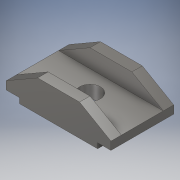
# Autodesk Inventor part: Block2
Saved by Autodesk Inventor 2019 (Build 230136000, 136)
## iProperties
Created: 2018-11-06
Part Number: Block2
Material: Stainless Steel
Document SubType Name: Modeling
Designer: 2003189
Density: 8 g/cm^3
Appearance: Semi-Polished
Mass: 1331.26 g
Surface Area: 349.634 cm^2
Volume: 166.407 cm^3
Author: 2003189
Autodesk Inventor part; units mm, degrees
ref_plane "YZ Plane" through (0, 0, 0) normal (1, 0, 0) x (0, 1, 0)
ref_plane "XZ Plane" through (0, 0, 0) normal (0, 1, 0) x (-1, 0, 0)
ref_plane "XY Plane" through (0, 0, 0) normal (0, 0, 1) x (1, 0, 0)
sketch "Sketch1" plane through (0, 0, 0) normal (0, 0, 1) x (1, 0, 0)
  line L0 (0, 0) -> (127, 0)
  line L1 (127, 0) -> (127, 38.1)
  line L2 (127, 38.1) -> (0, 38.1)
  line L3 (0, 38.1) -> (0, 0)
  line L4 (0, 0) -> (16.129, 0)
  line L5 (127, 0) -> (110.871, 0)
  line L6 (16.129, 0) -> (16.129, 6.35)
  line L7 (16.129, 6.35) -> (0, 6.35)
  line L8 (110.871, 0) -> (110.871, 6.35)
  line L9 (110.871, 6.35) -> (127, 6.35)
  dimension "d0" = 127
  dimension "d1" = 38.1
  dimension "d2" = 16.129
  dimension "d3" = 16.129
  dimension "d4" = 6.35
  dimension "d5" = 6.35
  constraints: 20 end point, 6 point on line, 2 parallel, 2 perpendicular, 1 horizontal, 1 vertical
  measures "d0" distance of L2.end L1.end
  measures "d1" distance of L1.end L0.end
  measures "d2" distance of L0.start L4.end
  measures "d3" distance of L0.end L5.end
  measures "d4" distance of L4.end L6.end
  measures "d5" distance of L5.end L8.end
extrude "Extrusion1" add sketch "Sketch1" along normal blind 76.2 contours L6 L7 L3 L2 L1 L9 L8 L0
chamfer "Chamfer5" distance 38.1 angle 30 2 edges at (127, 38.1, 38.1) (0, 38.1, 38.1) measured on face at (126.5, 38.1, 38.1) measured on face at (0.5, 38.1, 38.1)
ref_plane "Work Plane1" through (88.9, 38.1, 0) normal (-1, 0, 0) x (0, 0, 1)
sketch "Sketch8" plane through (127, 6.35, 76.2) normal (1, 0, 0) x (0, 0, -1)
  line L0 (0, 0) -> (0, 9.753) projected
  line L1 (0, 9.753) -> (12.7, 9.753)
  line L2 (0, 9.753) -> (76.2, 9.753) projected
  line L3 (76.2, 9.753) -> (63.5, 9.753)
  line L4 (76.2, 31.75) -> (0, 31.75) projected
  line L5 (0, 9.753) -> (0, 106.4603)
  line L6 (63.5, 9.753) -> (63.5, 86.1683)
  line L7 (63.5, 86.1683) -> (0, 90.6953)
  line L8 (12.7, 9.753) -> (12.7, 89.7899)
  point P0 (76.2, -6.35)
  dimension "d35" = 12.7
  dimension "d36" = 12.7
  constraints: 12 end point, 4 point on line, 3 vertical
  measures "d35" distance of L0.end L1.end
  measures "d36" distance of L2.end L3.end
extrude "Extrusion5" cut sketch "Sketch8" against normal blind 254 contours L8 L4 L6 L2 | L8 L7 L6 L4
sketch "Sketch9" plane through (127, 16.103, 63.5) normal (0, 1, 0) x (1, 0, 0)
  line L0 (-127, 50.8) -> (-127, 0) projected
  line L1 (0, 0) -> (-127, 0) projected
  line L2 (0, 0) -> (0, 50.8) projected
  line L3 (0, 50.8) -> (-127, 50.8) projected
  line L4 (-38.1, 0) -> (-88.9, 0) projected
  circle A0 centre (-63.5, 25.4) radius 12.7
  point P0 (-127, 63.5)
  dimension "d40" = 25.4
  constraints: 1 centre point
  measures "d40" diameter of A0
extrude "Extrusion6" cut sketch "Sketch9" against normal blind 254 contours A0
body "Solid1"
